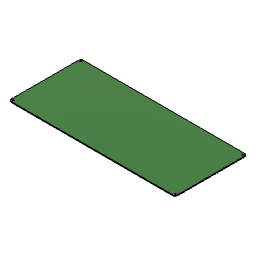
keyboard-v27-PCB-Placeholder (Autodesk Fusion 360 design; units mm, degrees)
Autodesk Fusion 360 part; units mm, degrees
sketch "Sketch1" plane through (0, 0, 0) normal (0, 0, 1) x (1, 0, 0)
  circle A0 centre (4.0951, 130.313) radius 1.5
  line L0 (3.5498, 134.069) -> (3.9274, 134.175)
  line L1 (2.4819, 133.578) -> (2.825, 133.769)
  line L2 (2.1566, 133.358) -> (2.4819, 133.578)
  line L3 (0.2329, 130.481) -> (0.339, 130.859)
  line L4 (3.1819, 133.933) -> (3.5498, 134.069)
  line L5 (1.0501, 132.252) -> (1.2926, 132.56)
  line L6 (4.7019, 134.298) -> (5.096, 134.313)
  line L7 (2.825, 133.769) -> (3.1819, 133.933)
  line L8 (0.1571, 130.096) -> (0.2329, 130.481)
  line L9 (4.3119, 134.251) -> (4.7019, 134.298)
  line L10 (1.5599, 132.848) -> (1.8479, 133.116)
  line L11 (1.2926, 132.56) -> (1.5599, 132.848)
  line L12 (0.339, 130.859) -> (0.4754, 131.226)
  line L13 (1.848, 133.116) -> (2.1566, 133.358)
  line L14 (0.831, 131.927) -> (1.0501, 132.252)
  line L15 (0.4754, 131.226) -> (0.6394, 131.583)
  line L16 (0.1102, 129.707) -> (0.1571, 130.096)
  line L17 (3.9274, 134.175) -> (4.3119, 134.251)
  line L18 (310.1945, 129.3093) -> (310.1945, 5.3108)
  line L19 (0.6394, 131.583) -> (0.831, 131.927)
  line L20 (0.0951, 129.312) -> (0.1102, 129.707)
  line L21 (306.361, 0.4534) -> (305.977, 0.3762)
  line L22 (305.587, 0.3294) -> (305.194, 0.3142)
  circle A1 centre (306.1945, 4.3142) radius 1.5
  line L23 (310.056, 4.1465) -> (309.95, 3.7689)
  line L24 (310.1945, 5.3108) -> (310.1774, 4.9174)
  line L25 (310.1774, 4.9174) -> (310.133, 4.5324)
  line L26 (1.0501, 2.3757) -> (0.831, 2.7023)
  line L27 (3.1819, 0.6945) -> (2.825, 0.8585)
  line L28 (0.2329, 4.1465) -> (0.1571, 4.5324)
  line L29 (0.831, 2.7023) -> (0.6394, 3.0455)
  line L30 (0.339, 3.7689) -> (0.2329, 4.1465)
  line L31 (1.848, 1.5117) -> (1.5599, 1.7791)
  line L32 (3.9274, 0.4534) -> (3.5498, 0.5595)
  line L33 (0.1571, 4.5324) -> (0.1102, 4.9223)
  line L34 (0.4754, 3.401) -> (0.339, 3.7689)
  circle A2 centre (4.0951, 4.3142) radius 1.5
  line L35 (305.194, 0.3142) -> (5.096, 0.3142)
  line L36 (310.133, 4.5324) -> (310.056, 4.1465)
  line L37 (309.24, 2.3757) -> (308.996, 2.0671)
  line L38 (2.4819, 1.0514) -> (2.1566, 1.2692)
  line L39 (2.1566, 1.2692) -> (1.8479, 1.5117)
  line L40 (308.73, 1.7791) -> (308.442, 1.5117)
  line L41 (307.807, 1.0514) -> (307.464, 0.8585)
  line L42 (307.464, 0.8585) -> (307.107, 0.6945)
  line L43 (2.825, 0.8585) -> (2.4819, 1.0514)
  line L44 (309.649, 3.0455) -> (309.458, 2.7023)
  line L45 (306.739, 0.5595) -> (306.361, 0.4534)
  line L46 (3.5498, 0.5595) -> (3.1819, 0.6945)
  line L47 (0.6394, 3.0455) -> (0.4754, 3.401)
  line L48 (4.7019, 0.3294) -> (4.3119, 0.3762)
  line L49 (308.132, 1.2692) -> (307.807, 1.0514)
  line L50 (307.107, 0.6945) -> (306.739, 0.5595)
  line L51 (4.3119, 0.3762) -> (3.9274, 0.4534)
  line L52 (1.2926, 2.0671) -> (1.0501, 2.3757)
  line L53 (308.996, 2.0671) -> (308.73, 1.7791)
  line L54 (308.442, 1.5117) -> (308.132, 1.2692)
  line L55 (309.458, 2.7023) -> (309.24, 2.3757)
  line L56 (308.132, 133.358) -> (308.442, 133.116)
  line L57 (305.977, 134.251) -> (306.361, 134.175)
  line L58 (5.096, 134.313) -> (305.194, 134.313)
  line L59 (77.0546, 0.3142) -> (190.5635, 0.3142)
  line L60 (0.0951, 5.3151) -> (0.0951, 129.312)
  line L61 (307.464, 133.769) -> (307.807, 133.578)
  line L62 (305.587, 134.298) -> (305.977, 134.251)
  line L63 (305.194, 134.313) -> (305.587, 134.298)
  line L64 (310.1786, 129.702) -> (310.1945, 129.3093)
  line L65 (307.107, 133.933) -> (307.464, 133.769)
  line L66 (306.739, 134.069) -> (307.107, 133.933)
  line L67 (308.996, 132.56) -> (309.24, 132.252)
  line L68 (310.056, 130.481) -> (310.133, 130.096)
  line L69 (309.24, 132.252) -> (309.458, 131.927)
  circle A3 centre (306.1945, 130.313) radius 1.5
  line L70 (310.133, 130.096) -> (310.1786, 129.702)
  line L71 (309.813, 131.226) -> (309.95, 130.859)
  line L72 (308.442, 133.116) -> (308.73, 132.848)
  line L73 (307.807, 133.578) -> (308.132, 133.358)
  line L74 (306.361, 134.175) -> (306.739, 134.069)
  line L75 (309.95, 130.859) -> (310.056, 130.481)
  line L76 (309.649, 131.583) -> (309.813, 131.226)
  line L77 (309.458, 131.927) -> (309.649, 131.583)
  line L78 (308.73, 132.848) -> (308.996, 132.56)
  line L79 (309.813, 3.401) -> (309.649, 3.0455)
  line L80 (0.1102, 4.9223) -> (0.0951, 5.3151)
  line L81 (5.096, 0.3142) -> (4.7019, 0.3294)
  line L82 (1.5599, 1.7791) -> (1.2926, 2.0671)
  line L83 (309.95, 3.7689) -> (309.813, 3.401)
  line L84 (305.977, 0.3762) -> (305.587, 0.3294)
  line L85 (189.7195, 134.313) -> (175.4705, 134.313)
  line L86 (175.4705, 134.313) -> (175.4705, 119.313)
  line L87 (175.4705, 119.313) -> (189.7195, 119.313)
  line L88 (189.7195, 119.313) -> (189.7195, 134.313)
  line L89 (162.5451, 119.783) -> (142.1051, 119.783)
  line L90 (142.1051, 119.783) -> (142.1051, 124.983)
  line L91 (142.1051, 124.983) -> (162.5451, 124.983)
  line L92 (162.5451, 124.983) -> (162.5451, 119.783)
  line L93 (172.0551, 119.923) -> (164.3351, 119.923)
  line L94 (164.3351, 119.923) -> (164.3351, 127.923)
  line L95 (164.3351, 127.923) -> (172.0551, 127.923)
  line L96 (172.0551, 127.923) -> (172.0551, 119.923)
  dimension "d381" = 3
  dimension "d382" = 3
  dimension "d383" = 3
  dimension "d384" = 3
  dimension "d385" = 4
  dimension "d386" = 4
  dimension "d387" = 4
  dimension "d388" = 4
  dimension "d389" = 4
  dimension "d390" = 4
  dimension "d391" = 4
  dimension "d392" = 4
  dimension "d414" = 123.9985
  dimension "d415" = 300.098
  dimension "d582" = 14.249
  dimension "d583" = 15
  dimension "d584" = 120.475
  dimension "d585" = 20.44
  dimension "d586" = 5.2
  dimension "d587" = 142.01
  dimension "d588" = 9.33
  dimension "d589" = 8
  dimension "d590" = 7.72
  dimension "d591" = 1.79
  dimension "d592" = 6.39
  constraint horizontal L35
  constraint horizontal L59
  constraint coincident L59.start L35
  constraint horizontal L85
  constraint vertical L86
  constraint horizontal L87
  constraint vertical L88
  constraint coincident L58 L85.start
  constraint horizontal L89
  constraint vertical L90
  constraint horizontal L91
  constraint vertical L92
  constraint horizontal L93
  constraint vertical L94
  constraint horizontal L95
  constraint vertical L96
  measures "d381" diameter of A2
  measures "d382" diameter of A0
  measures "d383" diameter of A3
  measures "d384" diameter of A1
  measures "d385" horizontal distance of L60.start A2.centre
  measures "d386" distance of A2.centre L35
  measures "d387" distance of A0.centre L60
  measures "d388" distance of A0.centre L58
  measures "d389" distance of A3.centre L18
  measures "d390" distance of A3.centre L58
  measures "d391" distance of A1.centre L18
  measures "d392" distance of A1.centre L35
  measures "d414" distance of L18.start L18.end
  measures "d415" distance of L22.end L35.end
  measures "d582" distance of L86.end L87.end
  measures "d583" distance of L85.start L87.end
  measures "d584" distance of L18 L88
  measures "d585" distance of L90.end L91.end
  measures "d586" distance of L89.start L91.end
  measures "d587" distance of L60 L90
  measures "d588" distance of L58 L91
  measures "d589" distance of L93.start L95.end
  measures "d590" distance of L93.start L93.end
  measures "d591" distance of L92 L94
  measures "d592" distance of L58 L95
extrude "Extrude1" add sketch "Sketch1" along normal blind 1.6 contours L0 L1 L2 L3 L4 L5 L6 L7 L8 L9 L10 L11 L12 L13 L14 L15 L16 L17 L18 L19 L20 L21 L22 L23 L24 L25 L26 L27 L28 L29 L30 L31 L32 L33 L34 L35 L36 L37 L38 L39 L40 L41 L42 L43 L44 L45 L46 L47 L48 L49 L50 L51 L52 L53 L54 L55 L56 L57 L58 L59 L60 L61 L62 L63 L64 L65 L66 L67 L68 L69 L70 L71 L72 L73 L74 L75 L76 L77 L78 L79 L80 L81 L82 L83 L84 L86 L87 L88 | L58 L85 L86 L87 L88 | L89 L90 L91 L92 | L93 L94 L95 L96
